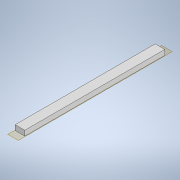
# Autodesk Inventor part: ferrite_bar_long
Saved by Autodesk Inventor 2020 (Build 240168000, 168)
## iProperties
Created: 2021-02-02
Part Number: ferrite_bar_long
Material: Generic
Document SubType Name: Modeling
Designer: phamv
Density: 1 g/cm^3
Appearance: Default
Author: phamv
Autodesk Inventor part; units mm, degrees
ref_plane "YZ Plane" through (0, 0, 0) normal (1, 0, 0) x (0, 1, 0)
ref_plane "XY Plane" through (0, 0, 0) normal (0, 0, 1) x (1, 0, 0)
sketch "Sketch1" plane through (0, 0, 0) normal (0, 1, 0) x (-1, 0, 0)
  line L0 (0, 109) -> (15, 109)
  line L1 (15, 109) -> (15, -109)
  line L2 (15, -109) -> (0, -109)
  line L3 (0, -109) -> (0, 109)
  point P0 (0, 0)
  point P1 (0, 0)
  dimension "d0" = 218
  dimension "d1" = 15
  constraints: 8 end point, 2 parallel, 1 coincident, 1 horizontal, 1 midpoint, 1 perpendicular
  measures "d0" distance between parallel lines of L2 L0
  measures "d1" distance between parallel lines of L1 L3
extrude "Extrusion1" add sketch "Sketch1" along normal blind 8
equation "\"d0\" = ferrite_length"
equation "\"d1\" = ferrite_width"
equation "\"d2\" = ferrite_height"
equation "\"ferrite_length\" = 218"
equation "\"ferrite_width\" = 15"
equation "\"ferrite_height\" = 8"
body "Solid1"
